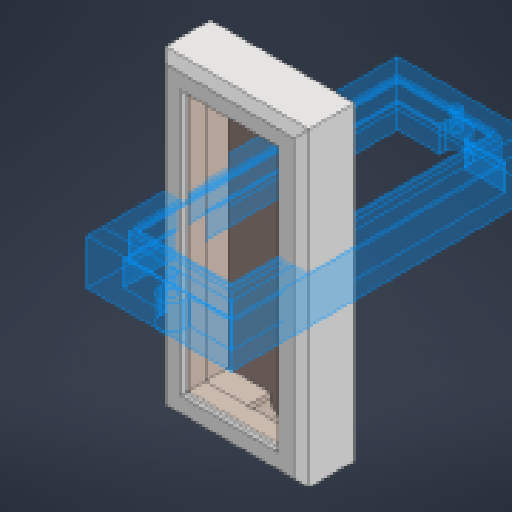
# Autodesk Inventor part: flat base
Saved by Autodesk Inventor 2024.3 (Build 283343000, 343)
## iProperties
Created: 2025-08-06
Part Number: flat base
Material: Generic
Document SubType Name: Modeling
Designer: giuseppe
Density: 1 g/cm^3
Appearance: Default
Author: giuseppe
Autodesk Inventor part; units mm, degrees
ref_plane "YZ Plane" through (0, 0, 0) normal (1, 0, 0) x (0, 1, 0)
ref_plane "XZ Plane" through (0, 0, 0) normal (0, 1, 0) x (-1, 0, 0)
ref_plane "XY Plane" through (0, 0, 0) normal (0, 0, 1) x (1, 0, 0)
ref_plane "Work Plane1" through (0, 0, 0) normal (0, 0, 1) x (1, 0, 0)
sketch "Sketch1" plane through (0, 0, 0) normal (0, 0, 1) x (1, 0, 0)
  line L0 (2, -8.6027) -> (2, -14.75) construction
  line L1 (2, -14.75) -> (-17, -5.2524) construction
  line L2 (-17, -5.2524) -> (-2, -7.8973) construction
  line L3 (-2, -7.8973) -> (-2, -1.75) construction
  line L4 (-2, -1.75) -> (17, -11.2476) construction
  line L5 (17, -11.2476) -> (2, -8.6027) construction
  line L6 (2, 40.8973) -> (2, 34.75) construction
  line L7 (2, 34.75) -> (-17, 44.2476) construction
  line L8 (-17, 44.2476) -> (-2, 41.6027) construction
  line L9 (-2, 41.6027) -> (-2, 47.75) construction
  line L10 (-2, 47.75) -> (17, 38.2524) construction
  line L11 (17, 38.2524) -> (2, 40.8973) construction
  line L12 (2, -25.1027) -> (2, -31.25) construction
  line L13 (2, -31.25) -> (-17, -21.7524) construction
  line L14 (-17, -21.7524) -> (-2, -24.3973) construction
  line L15 (-2, -24.3973) -> (-2, -18.25) construction
  line L16 (-2, -18.25) -> (17, -27.7476) construction
  line L17 (17, -27.7476) -> (2, -25.1027) construction
  line L18 (2, 7.8973) -> (2, 1.75) construction
  line L19 (2, 1.75) -> (-17, 11.2476) construction
  line L20 (-17, 11.2476) -> (-2, 8.6027) construction
  line L21 (-2, 8.6027) -> (-2, 14.75) construction
  line L22 (-2, 14.75) -> (17, 5.2524) construction
  line L23 (17, 5.2524) -> (2, 7.8973) construction
  line L24 (2, 24.3973) -> (2, 18.25) construction
  line L25 (2, 18.25) -> (-17, 27.7476) construction
  line L26 (-17, 27.7476) -> (-2, 25.1027) construction
  line L27 (-2, 25.1027) -> (-2, 31.25) construction
  line L28 (-2, 31.25) -> (17, 21.7524) construction
  line L29 (17, 21.7524) -> (2, 24.3973) construction
  line L30 (2, -41.6027) -> (2, -47.75) construction
  line L31 (2, -47.75) -> (-17, -38.2524) construction
  line L32 (-17, -38.2524) -> (-2, -40.8973) construction
  line L33 (-2, -40.8973) -> (-2, -34.75) construction
  line L34 (-2, -34.75) -> (17, -44.2476) construction
  line L35 (17, -44.2476) -> (2, -41.6027) construction
  line L36 (-20, 52.75) -> (-20, -52.75) construction
  line L37 (-20, -52.75) -> (20, -52.75) construction
  line L38 (20, -52.75) -> (20, 52.75) construction
  line L39 (20, 52.75) -> (-20, 52.75) construction
  line L40 (18.5, 51.55) -> (-18.5, 51.55)
  line L41 (-18.5, 51.55) -> (-18.5, -51.25)
  line L42 (-18.5, -51.25) -> (18.5, -51.25)
  line L43 (18.5, -51.25) -> (18.5, 51.55)
  line L44 (28.5, 61.55) -> (-28.5, 61.55)
  line L45 (-28.5, 61.55) -> (-28.5, -61.25)
  line L46 (-28.5, -61.25) -> (28.5, -61.25)
  line L47 (28.5, -61.25) -> (28.5, 61.55)
  point P0 (0, 0)
  dimension "d0" = 1.5
  dimension "d1" = 1.2
  dimension "d2" = 1.5
  dimension "d3" = 1.5
  dimension "d4" = 10
  dimension "d5" = 10
  dimension "d6" = 10
  dimension "d7" = 10
  constraints: 16 end point, 4 parallel, 2 horizontal, 2 perpendicular
  measures "d0" distance between parallel lines of L38 L43
  measures "d1" distance between parallel lines of L39 L40
  measures "d2" distance between parallel lines of L36 L41
  measures "d3" distance between parallel lines of L37 L42
  measures "d4" distance between parallel lines of L46 L42
  measures "d5" distance between parallel lines of L40 L44
  measures "d6" distance between parallel lines of L47 L43
  measures "d7" distance between parallel lines of L41 L45
extrude "Extrusion1" add sketch "Sketch1" along normal blind 2
sketch "Sketch2" plane through (0, 0, 0) normal (0, 0, -1) x (-1, 0, 0)
  line L0 (-17, 38.2524) -> (2, 47.75) construction
  line L1 (2, 47.75) -> (2, 41.6027) construction
  line L2 (2, 41.6027) -> (17, 44.2476) construction
  line L3 (17, 44.2476) -> (-2, 34.75) construction
  line L4 (-2, 34.75) -> (-2, 40.8973) construction
  line L5 (-2, 40.8973) -> (-17, 38.2524) construction
  line L6 (-17, 21.7524) -> (2, 31.25) construction
  line L7 (2, 31.25) -> (2, 25.1027) construction
  line L8 (2, 25.1027) -> (17, 27.7476) construction
  line L9 (17, 27.7476) -> (-2, 18.25) construction
  line L10 (-2, 18.25) -> (-2, 24.3973) construction
  line L11 (-2, 24.3973) -> (-17, 21.7524) construction
  line L12 (-17, 5.2524) -> (2, 14.75) construction
  line L13 (2, 14.75) -> (2, 8.6027) construction
  line L14 (2, 8.6027) -> (17, 11.2476) construction
  line L15 (17, 11.2476) -> (-2, 1.75) construction
  line L16 (-2, 1.75) -> (-2, 7.8973) construction
  line L17 (-2, 7.8973) -> (-17, 5.2524) construction
  line L18 (-17, -11.2476) -> (2, -1.75) construction
  line L19 (2, -1.75) -> (2, -7.8973) construction
  line L20 (2, -7.8973) -> (17, -5.2524) construction
  line L21 (17, -5.2524) -> (-2, -14.75) construction
  line L22 (-2, -14.75) -> (-2, -8.6027) construction
  line L23 (-2, -8.6027) -> (-17, -11.2476) construction
  line L24 (-17, -27.7476) -> (2, -18.25) construction
  line L25 (2, -18.25) -> (2, -24.3973) construction
  line L26 (2, -24.3973) -> (17, -21.7524) construction
  line L27 (17, -21.7524) -> (-2, -31.25) construction
  line L28 (-2, -31.25) -> (-2, -25.1027) construction
  line L29 (-2, -25.1027) -> (-17, -27.7476) construction
  line L30 (-17, -44.2476) -> (2, -34.75) construction
  line L31 (2, -34.75) -> (2, -40.8973) construction
  line L32 (2, -40.8973) -> (17, -38.2524) construction
  line L33 (17, -38.2524) -> (-2, -47.75) construction
  line L34 (-2, -47.75) -> (-2, -41.6027) construction
  line L35 (-2, -41.6027) -> (-17, -44.2476) construction
  line L36 (20, 52.75) -> (20, -52.75) construction
  line L37 (-20, 52.75) -> (20, 52.75) construction
  line L38 (-20, -52.75) -> (-20, 52.75) construction
  line L39 (20, -52.75) -> (-20, -52.75) construction
  line L40 (-20.5, -53.25) -> (20.5, -53.25)
  line L41 (20.5, -53.25) -> (20.5, 53.25)
  line L42 (20.5, 53.25) -> (-20.5, 53.25)
  line L43 (-20.5, 53.25) -> (-20.5, -53.25)
  line L44 (28.5, 61.55) -> (28.5, -61.25) projected
  line L45 (-28.5, 61.55) -> (28.5, 61.55) projected
  line L46 (-28.5, -61.25) -> (-28.5, 61.55) projected
  line L47 (28.5, -61.25) -> (-28.5, -61.25) projected
  line L48 (-18.5, 51.55) -> (-18.5, -51.25) projected
  line L49 (18.5, 51.55) -> (-18.5, 51.55) projected
  line L50 (18.5, -51.25) -> (18.5, 51.55) projected
  line L51 (-18.5, -51.25) -> (18.5, -51.25) projected
  dimension "d10" = 0.5
  dimension "d11" = 0.5
  dimension "d12" = 0.5
  dimension "d13" = 0.5
  constraints: 8 end point, 2 parallel, 1 horizontal, 1 perpendicular
  measures "d10" distance between parallel lines of L43 L38
  measures "d11" distance between parallel lines of L40 L39
  measures "d12" distance between parallel lines of L36 L41
  measures "d13" distance between parallel lines of L42 L37
ref_plane "Work Plane2" through (-20, -52.75, -3) normal (0, 0, -1) x (0, 1, 0)
extrude "Extrusion2" add sketch "Sketch2" along normal up to surface (3 mm away) contours L44 L47 L46 L45
sketch "Sketch3" plane through (28.5, 61.55, -3) normal (0, 0, -1) x (-1, 0, 0)
  line L0 (8, -114.8) -> (49, -114.8) projected
  line L1 (8, -8.3) -> (8, -114.8) projected
  line L2 (49, -8.3) -> (8, -8.3) projected
  line L3 (49, -114.8) -> (49, -8.3) projected
  line L4 (0, 0) -> (57, 0) projected
  line L5 (0, -122.8) -> (0, 0) projected
  line L6 (57, -122.8) -> (0, -122.8) projected
  line L7 (57, 0) -> (57, -122.8) projected
  point P0 (28.5, -61.55)
ref_plane "Work Plane3" through (-20.5, -60, -9) normal (0, 0, 1) x (1, 0, 0)
extrude "Extrusion3" add sketch "Sketch3" along normal up to surface (6 mm away)
sketch "Sketch4" plane through (28.5, -61.25, -9) normal (0, 0, -1) x (-1, 0, 0)
  circle A0 centre (28.5, 5) radius 1.75 projected
  circle A1 centre (28.5, 117.8) radius 1.75 projected
  point P0 (28.5, 61.25)
hole "Hole1" at (0, -56.25, -9) at (0, 56.55, -9) direction (0, 0, 1) diameter 3.7 depth 7
sketch "Sketch5" plane through (28.5, -61.25, -9) normal (0, 0, -1) x (-1, 0, 0)
  circle A0 centre (28.5, 5) radius 1.75 projected
  line L0 (8, 114.5) -> (8, 8) projected
  line L1 (8, 8) -> (24.75, 8) projected
  line L2 (24.75, 8) -> (24.75, 5) projected
  arc A1 (24.75, 5) -> (32.25, 5) centre (28.5, 5) ccw projected
  line L3 (32.25, 5) -> (32.25, 8) projected
  line L4 (32.25, 8) -> (49, 8) projected
  line L5 (49, 8) -> (49, 114.5) projected
  line L6 (49, 114.5) -> (8, 114.5) projected
  line L7 (23.75, 7) -> (7, 7)
  line L8 (7, 7) -> (7, 115.5)
  line L9 (7, 115.5) -> (50, 115.5)
  line L10 (50, 115.5) -> (50, 7)
  line L11 (50, 7) -> (33.25, 7)
  line L12 (33.25, 7) -> (33.25, 5)
  arc A2 (23.75, 5) -> (33.25, 5) centre (28.5, 5) ccw
  line L13 (23.75, 5) -> (23.75, 7)
  circle A3 centre (28.5, 117.8) radius 1.85 projected
  circle A4 centre (28.5, 5) radius 1.85 projected
  line L14 (49, 8) -> (8, 8) projected
  line L15 (8, 8) -> (8, 114.5) projected
  line L16 (8, 114.5) -> (49, 114.5) projected
  line L17 (49, 114.5) -> (49, 8) projected
  line L18 (0, 122.8) -> (0, 0) projected
  line L19 (0, 0) -> (57, 0) projected
  line L20 (57, 0) -> (57, 122.8) projected
  line L21 (57, 122.8) -> (0, 122.8) projected
  circle A5 centre (28.5, 117.8) radius 1.75 projected
  line L22 (32.25, 117.8) -> (32.25, 114.8) projected
  arc A6 (32.25, 117.8) -> (24.75, 117.8) centre (28.5, 117.8) ccw projected
  line L23 (24.75, 114.8) -> (24.75, 117.8) projected
  line L24 (32.25, 114.8) -> (24.75, 114.8) projected
  circle A7 centre (28.5, 117.8) radius 1.75 projected
  arc A8 (33.25, 117.8) -> (23.75, 117.8) centre (28.5, 117.8) ccw
  line L25 (33.25, 117.8) -> (33.25, 113.8)
  line L26 (33.25, 113.8) -> (23.75, 113.8)
  line L27 (23.75, 113.8) -> (23.75, 117.8)
  point P0 (28.5, 61.25)
  point P1 (23.75, 115.5)
  point P2 (33.25, 115.5)
  dimension "d25" = 1
  dimension "d26" = 1
  constraints: 20 end point, 4 point on circle, 2 centre point, 10 other
  measures "d25" distance between parallel lines of L1 L7
  measures "d26" radial gap between concentric circles of A6 A8
extrude "Extrusion4" add sketch "Sketch5" along normal blind 10 contours L21 L20 L19 L18
chamfer "Chamfer1" distance 3 angle 45 4 edges at (-28.5, 0.15, 2) (0, 61.55, 2) (28.5, 0.15, 2) (0, -61.25, 2)
chamfer "Chamfer2" distance 1 angle 45 4 edges at (-18.5, 0.15, 2) (0, -51.25, 2) (0, 51.55, 2) (18.5, 0.15, 2)
body "Solid1"
